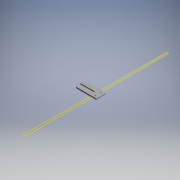
# Autodesk Inventor part: Idler
Saved by Autodesk Inventor 2018 (Build 220112000, 112)
## iProperties
Created: 2018-05-19
Part Number: Idler
Material: Generic
Document SubType Name: Modeling
Designer: dan
Density: 1 g/cm^3
Appearance: Default
Author: dan
Autodesk Inventor part; units mm, degrees
ref_plane "YZ Plane" through (0, 0, 0) normal (1, 0, 0) x (0, 1, 0)
ref_plane "XZ Plane" through (0, 0, 0) normal (0, 1, 0) x (-1, 0, 0)
ref_plane "XY Plane" through (0, 0, 0) normal (0, 0, 1) x (1, 0, 0)
ref_plane "Work Plane1" through (0, 0, 0) normal (0, 0, 1) x (1, 0, 0)
sketch "Sketch1" plane through (0, 0, 0) normal (0, 0, 1) x (1, 0, 0)
  line L0 (27.9999, -0.0002) -> (27.9999, 599.9998) projected
  line L1 (-2, -0.0002) -> (-2, 599.9998) projected
  line L2 (-75.0445, 277.7834) -> (27.9999, 277.7834)
  line L3 (27.9999, 277.7834) -> (27.9999, 322.2162)
  line L4 (27.9999, 322.2162) -> (-75.0445, 322.2162)
  line L5 (-75.0445, 322.2162) -> (-75.0445, 277.7834)
  line L6 (-75.0445, 277.7834) -> (27.9999, 322.2162) construction
  line L7 (27.9999, 277.7834) -> (-75.0445, 322.2162) construction
  line L8 (-5.6506, 302.4998) -> (-67.1503, 302.4998)
  line L9 (-66.9479, 297.5039) -> (-5.7013, 297.5039)
  line L10 (-5.6506, 302.4998) -> (-66.9479, 297.5039) construction
  line L11 (-67.1503, 302.4998) -> (-5.7013, 297.5039) construction
  arc A0 (-67.1503, 302.4998) -> (-66.9479, 297.5039) centre (-67.3544, 299.9894) ccw
  arc A1 (-5.7013, 297.5039) -> (-5.9109, 302.4785) centre (-5.578, 300.0008) ccw
  line L12 (27.9999, 277.7834) -> (12.9999, 277.7834)
  circle A2 centre (12.9999, 287.7834) radius 2.5
  circle A3 centre (12.9999, 312.2162) radius 2.5
  line L13 (12.9999, 277.7834) -> (12.9999, 285.2834)
  point P0 (0, 0)
  point P1 (-23.5223, 299.9998)
  point P2 (-36.3624, 299.9967)
  dimension "d4" = 5
  dimension "d0" = 5
  dimension "d1" = 15
  dimension "d5" = 5
  constraints: 25 end point, 5 point on circle, 5 point on line, 3 centre point, 3 parallel, 2 horizontal, 2 midpoint, 2 perpendicular, 1 tangent, 1 vertical alignment, 2 other
  measures "d0" distance of L9.start L8.end
  measures "d1" distance of L2.end L12.end
  measures "d5" diameter of A3
extrude "Extrusion1" add sketch "Sketch1" along normal blind 6
fillet "Fillet1" radius 15 2 edges at (-75.0445, 277.7834, 3) (-75.0445, 322.2162, 3)
body "Solid1"
